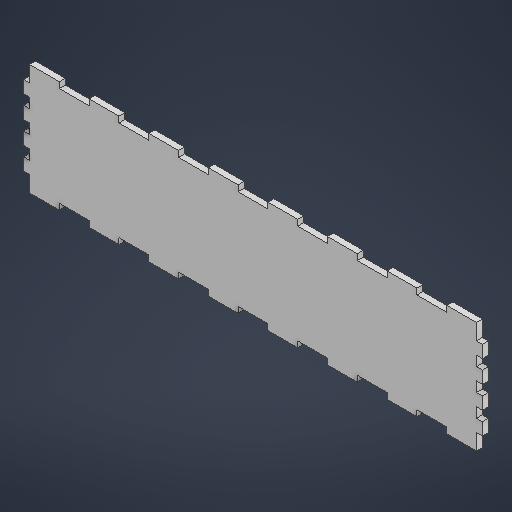
# Autodesk Inventor part: AnchoBase
Saved by Autodesk Inventor 2026 (Build 300175000, 175)
## iProperties
Created: 2026-04-21
Part Number: AnchoBase
Material: Generic
Document SubType Name: Modeling
Designer: juana
Density: 1 g/cm^3
Appearance: Default
Author: juana
Autodesk Inventor part; units mm, degrees
ref_plane "YZ Plane" through (0, 0, 0) normal (1, 0, 0) x (0, 1, 0)
ref_plane "XZ Plane" through (0, 0, 0) normal (0, 1, 0) x (-1, 0, 0)
ref_plane "XY Plane" through (0, 0, 0) normal (0, 0, 1) x (1, 0, 0)
sketch "Sketch1" plane through (0, 0, 0) normal (0, 0, 1) x (1, 0, 0)
  line L0 (0, 0) -> (225, 0)
  line L1 (225, 0) -> (225, 50)
  line L2 (225, 50) -> (0, 50)
  line L3 (0, 50) -> (0, 0)
  line L4 (-3, 45) -> (0, 45)
  line L5 (0, 45) -> (0, 38.75)
  line L6 (0, 38.75) -> (-3, 38.75)
  line L7 (-3, 38.75) -> (-3, 45)
  line L8 (0, 0) -> (15, 0)
  line L9 (15, 0) -> (15, -3)
  line L10 (15, -3) -> (0, -3)
  line L11 (0, -3) -> (0, 0)
  line L12 (-3, 33.75) -> (0, 33.75)
  line L13 (0, 33.75) -> (0, 27.5)
  line L14 (-3, 27.5) -> (-3, 33.75)
  line L15 (0, 27.5) -> (-3, 27.5)
  line L16 (-3, 22.5) -> (0, 22.5)
  line L17 (0, 22.5) -> (0, 16.25)
  line L18 (-3, 16.25) -> (-3, 22.5)
  line L19 (0, 16.25) -> (-3, 16.25)
  line L20 (-3, 11.25) -> (0, 11.25)
  line L21 (0, 11.25) -> (0, 5)
  line L22 (-3, 5) -> (-3, 11.25)
  line L23 (0, 5) -> (-3, 5)
  line L24 (225, 45) -> (228, 45)
  line L25 (228, 45) -> (228, 38.75)
  line L26 (225, 38.75) -> (225, 45)
  line L27 (228, 38.75) -> (225, 38.75)
  line L28 (225, 33.75) -> (228, 33.75)
  line L29 (228, 33.75) -> (228, 27.5)
  line L30 (225, 27.5) -> (225, 33.75)
  line L31 (228, 27.5) -> (225, 27.5)
  line L32 (225, 22.5) -> (228, 22.5)
  line L33 (228, 22.5) -> (228, 16.25)
  line L34 (225, 16.25) -> (225, 22.5)
  line L35 (228, 16.25) -> (225, 16.25)
  line L36 (225, 11.25) -> (228, 11.25)
  line L37 (228, 11.25) -> (228, 5)
  line L38 (225, 5) -> (225, 11.25)
  line L39 (228, 5) -> (225, 5)
  line L40 (45, -3) -> (30, -3)
  line L41 (30, -3) -> (30, 0)
  line L42 (45, 0) -> (45, -3)
  line L43 (30, 0) -> (45, 0)
  line L44 (75, -3) -> (60, -3)
  line L45 (60, -3) -> (60, 0)
  line L46 (75, 0) -> (75, -3)
  line L47 (60, 0) -> (75, 0)
  line L48 (105, -3) -> (90, -3)
  line L49 (90, -3) -> (90, 0)
  line L50 (105, 0) -> (105, -3)
  line L51 (90, 0) -> (105, 0)
  line L52 (135, -3) -> (120, -3)
  line L53 (120, -3) -> (120, 0)
  line L54 (135, 0) -> (135, -3)
  line L55 (120, 0) -> (135, 0)
  line L56 (165, -3) -> (150, -3)
  line L57 (150, -3) -> (150, 0)
  line L58 (165, 0) -> (165, -3)
  line L59 (150, 0) -> (165, 0)
  line L60 (195, -3) -> (180, -3)
  line L61 (180, -3) -> (180, 0)
  line L62 (195, 0) -> (195, -3)
  line L63 (180, 0) -> (195, 0)
  line L64 (225, -3) -> (210, -3)
  line L65 (210, -3) -> (210, 0)
  line L66 (225, 0) -> (225, -3)
  line L67 (210, 0) -> (225, 0)
  line L68 (15, 50) -> (0, 50)
  line L69 (0, 50) -> (0, 53)
  line L70 (15, 53) -> (15, 50)
  line L71 (0, 53) -> (15, 53)
  line L72 (45, 50) -> (30, 50)
  line L73 (30, 50) -> (30, 53)
  line L74 (45, 53) -> (45, 50)
  line L75 (30, 53) -> (45, 53)
  line L76 (75, 50) -> (60, 50)
  line L77 (60, 50) -> (60, 53)
  line L78 (75, 53) -> (75, 50)
  line L79 (60, 53) -> (75, 53)
  line L80 (105, 50) -> (90, 50)
  line L81 (90, 50) -> (90, 53)
  line L82 (105, 53) -> (105, 50)
  line L83 (90, 53) -> (105, 53)
  line L84 (135, 50) -> (120, 50)
  line L85 (120, 50) -> (120, 53)
  line L86 (135, 53) -> (135, 50)
  line L87 (120, 53) -> (135, 53)
  line L88 (165, 50) -> (150, 50)
  line L89 (150, 50) -> (150, 53)
  line L90 (165, 53) -> (165, 50)
  line L91 (150, 53) -> (165, 53)
  line L92 (195, 50) -> (180, 50)
  line L93 (180, 50) -> (180, 53)
  line L94 (195, 53) -> (195, 50)
  line L95 (180, 53) -> (195, 53)
  line L96 (225, 50) -> (210, 50)
  line L97 (210, 50) -> (210, 53)
  line L98 (225, 53) -> (225, 50)
  line L99 (210, 53) -> (225, 53)
  point P0 (0, 38.75)
  point P1 (0, 50)
  dimension "d0" = 225
  dimension "d1" = 50
  dimension "d4" = 6.25
  dimension "d5" = 3
  dimension "d6" = 5
  dimension "d7" = 15
  dimension "d8" = 3
  dimension "d13" = 11.25
  dimension "d16" = 228
  dimension "d21" = 30
  dimension "d24" = 53
  constraints: 200 end point, 6 parallel, 5 horizontal, 3 perpendicular, 2 vertical, 1 vertical alignment, 176 other
  measures "d0" distance of L1.end L2.end
  measures "d1" distance of L0.end L1.end
  measures "d4" distance of L6.end L4.start
  measures "d5" distance of L4.start L4.end
  measures "d6" distance between parallel lines of L2 L4
  measures "d7" distance of L9.end L10.end
  measures "d8" distance of L8.end L9.end
  measures "d13" distance of L4.start L12.start
  measures "d16" distance of L4.start L24.start
  measures "d21" distance of L9.end L40.start
  measures "d24" distance of L9.end L68.start
extrude "Extrusion1" add sketch "Sketch1" along normal blind 3 contours L3 L2 L1 L0 | L23 L22 L20 L3 | L19 L18 L16 L3 | L15 L14 L12 L3 | L6 L7 L4 L3 | L1 L36 L37 L39 | L1 L32 L33 L35 | L1 L28 L29 L31 | L1 L24 L25 L27
extrude "Extrusion2" add sketch "Sketch1" along normal blind 3 contours L0 L9 L10 L11 | L0 L42 L40 L41 | L0 L46 L44 L45 | L0 L50 L48 L49 | L0 L54 L52 L53 | L69 L71 L70 L2 | L0 L58 L56 L57 | L73 L75 L74 L2 | L0 L62 L60 L61 | L77 L79 L78 L2 | L0 L66 L64 L65 | L81 L83 L82 L2 | L85 L87 L86 L2 | L89 L91 L90 L2 | L93 L95 L94 L2 | L97 L99 L98 L2
body "Solid1"
